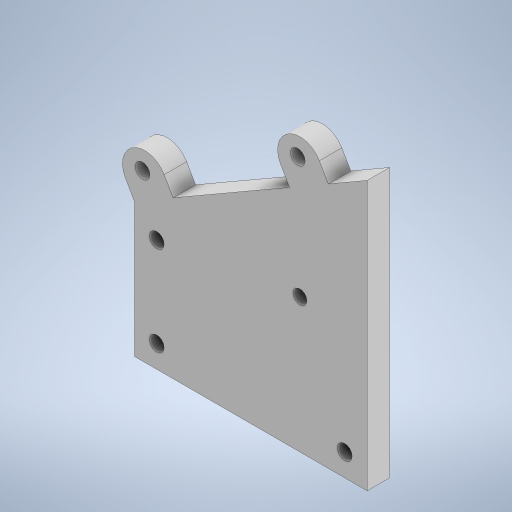
# Autodesk Inventor part: ベースパーツ1
Saved by Autodesk Inventor 2024.3 (Build 283343000, 343)
## iProperties
Created: 2024-10-08
Part Number: ベースパーツ1
Material: 一般
Document SubType Name: Modeling
Designer: hikou
Density: 1 g/cm^3
Appearance: 既定
Author: hikou
Autodesk Inventor part; units mm, degrees
ref_plane "YZ Plane" through (0, 0, 0) normal (1, 0, 0) x (0, 1, 0)
ref_plane "XZ Plane" through (0, 0, 0) normal (0, 1, 0) x (-1, 0, 0)
ref_plane "XY Plane" through (0, 0, 0) normal (0, 0, 1) x (1, 0, 0)
sketch "スケッチ1" plane through (0, 0, 0) normal (0, 0, 1) x (1, 0, 0)
  line L0 (-25.9808, -15) -> (25.9808, -15)
  line L1 (25.9808, -15) -> (25.9808, 15)
  line L2 (25.9808, 15) -> (-25.9808, 15)
  line L3 (-25.9808, 15) -> (-25.9808, -15)
  line L4 (-25.9808, -15) -> (25.9808, 15) construction
  line L5 (25.9808, -15) -> (-25.9808, 15) construction
  line L6 (-25.9808, 15) -> (25.9808, 45)
  line L7 (25.9808, 45) -> (25.9808, 15)
  line L8 (-25.9808, 15) -> (-30.9808, 23.6603)
  line L9 (-30.9808, 23.6603) -> (-22.3205, 28.6603)
  line L10 (-22.3205, 28.6603) -> (-17.3205, 20)
  line L11 (8.6603, 35) -> (3.6603, 43.6603)
  line L12 (3.6603, 43.6603) -> (12.3205, 48.6603)
  line L13 (12.3205, 48.6603) -> (17.3205, 40)
  point P0 (0, 0)
  dimension "d0" = 60
  dimension "d1" = 30
  dimension "d2" = 30
  dimension "d3" = 30
  dimension "d4" = 10
  dimension "d5" = 10
  dimension "d6" = 10
  dimension "d7" = 30
  constraints: 28 end point, 7 perpendicular, 4 point on line, 2 midpoint, 2 parallel, 1 horizontal
  measures "d0" distance of L2.end L6.end
  measures "d1" distance of L6.end L1.end
  measures "d2" angle of L2 L6
  measures "d3" distance of L0.end L1.end
  measures "d4" distance of L2.end L8.end
  measures "d5" distance of L8.end L9.end
  measures "d6" distance of L11.end L12.end
  measures "d7" distance between parallel lines of L10 L11
extrude "押し出し1" add sketch "スケッチ1" along normal mid plane 5
sketch "スケッチ2" plane through (0, 0, 2.5) normal (0, 0, 1) x (1, 0, 0)
  line L0 (-30.9808, 23.6603) -> (-25.9808, 15) projected
  line L1 (-25.9808, 15) -> (-25.9808, -15) projected
  line L2 (-25.9808, -15) -> (25.9808, -15) projected
  line L3 (25.9808, -15) -> (25.9808, 45) projected
  line L4 (25.9808, 45) -> (17.3205, 40) projected
  line L5 (17.3205, 40) -> (12.3205, 48.6603) projected
  line L6 (12.3205, 48.6603) -> (3.6603, 43.6603) projected
  line L7 (3.6603, 43.6603) -> (8.6603, 35) projected
  line L8 (8.6603, 35) -> (-17.3205, 20) projected
  line L9 (-17.3205, 20) -> (-22.3205, 28.6603) projected
  line L10 (-22.3205, 28.6603) -> (-30.9808, 23.6603) projected
  point P0 (0, 0)
  point P1 (-24.1506, 21.8301)
  point P2 (10.4904, 41.8301)
  dimension "d10" = 5
  dimension "d11" = 5
  dimension "d12" = 5
  dimension "d13" = 5
  measures "d10" distance from line of L8 point (-24.151, 21.83)
  measures "d11" distance from line of L8 point (10.49, 41.83)
  measures "d12" distance from line of L9 point (-24.151, 21.83)
  measures "d13" distance from line of point (10.49, 41.83) L7
hole "穴1" at (-24.1506, 21.8301, 2.5) at (10.4904, 41.8301, 2.5) direction (0, 0, -1) diameter 3.3 end through all
sketch "スケッチ3" plane through (0, 0, 2.5) normal (0, 0, 1) x (1, 0, 0)
  circle A0 centre (10.4904, 41.8301) radius 1.65 projected
  circle A1 centre (-24.1506, 21.8301) radius 1.65 projected
  line L0 (-30.9808, 23.6603) -> (-25.9808, 15) projected
  line L1 (-25.9808, 15) -> (-25.9808, -15) projected
  line L2 (-25.9808, -15) -> (25.9808, -15) projected
  line L3 (25.9808, -15) -> (25.9808, 45) projected
  line L4 (25.9808, 45) -> (17.3205, 40) projected
  line L5 (17.3205, 40) -> (12.3205, 48.6603) projected
  line L6 (12.3205, 48.6603) -> (3.6603, 43.6603) projected
  line L7 (3.6603, 43.6603) -> (8.6603, 35) projected
  line L8 (8.6603, 35) -> (-17.3205, 20) projected
  line L9 (-17.3205, 20) -> (-22.3205, 28.6603) projected
  line L10 (-22.3205, 28.6603) -> (-30.9808, 23.6603) projected
  circle A2 centre (-23.6506, 20.9641) radius 5
  circle A3 centre (10.9904, 40.9641) radius 5
  point P0 (0, 0)
  point P1 (6.6603, 38.4641)
  point P2 (15.3205, 43.4641)
  point P3 (-27.9808, 18.4641)
  point P4 (-19.3205, 23.4641)
  dimension "d21" = 10
  dimension "d22" = 1
  dimension "d24" = 4
  dimension "d25" = 10
  dimension "d26" = 1
  dimension "d27" = 4
  constraints: 2 centre point
  measures "d21" diameter of A2
  measures "d22" distance of A1.centre A2.centre
  measures "d24" distance from line of L8 A2.centre
  measures "d25" diameter of A3
  measures "d26" distance of A0.centre A3.centre
  measures "d27" distance from line of L8 A3.centre
extrude "押し出し2" cut sketch "スケッチ3" against normal blind 5 contours L10 L9 A2 L0 | L7 L6 L5 A3
sketch "スケッチ4" plane through (0, 0, 2.5) normal (0, 0, 1) x (1, 0, 0)
  line L0 (-25.9808, -15) -> (25.9808, -15) projected
  line L1 (25.9808, -15) -> (25.9808, 45) projected
  point P0 (0, 0)
  point P1 (10.9808, 15)
  dimension "d30" = 30
  dimension "d31" = 15
  measures "d30" distance from line of L0 point (10.981, 15)
  measures "d31" distance from line of L1 point (10.981, 15)
hole "穴2" at (10.9808, 15, 2.5) direction (0, 0, -1) diameter 3.1 end through all
sketch "スケッチ5" plane through (0, 0, 2.5) normal (0, 0, 1) x (1, 0, 0)
  line L0 (-25.9808, 15) -> (-25.9808, -15) projected
  line L1 (-25.9808, -15) -> (25.9808, -15) projected
  line L2 (25.9808, -15) -> (25.9808, 45) projected
  point P0 (0, 0)
  point P1 (-20.9808, 10)
  point P2 (-20.9808, -10)
  point P3 (20.9808, -10)
  dimension "d39" = 5
  dimension "d40" = 5
  dimension "d41" = 5
  dimension "d42" = 20
  dimension "d43" = 5
  dimension "d44" = 5
  measures "d39" distance from line of L0 point (-20.981, -10)
  measures "d40" distance from line of L1 point (-20.981, -10)
  measures "d41" distance from line of L0 point (-20.981, 10)
  measures "d42" distance of point (-20.981, -10) point (-20.981, 10)
  measures "d43" distance from line of L1 point (20.981, -10)
  measures "d44" distance from line of L2 point (20.981, -10)
hole "穴3" at (-20.9808, 10, 2.5) at (-20.9808, -10, 2.5) at (20.9808, -10, 2.5) direction (0, 0, -1) diameter 3.3 end through all
equation "\"d5\" = d4"
equation "\"d6\" = d4"
equation "\"d11\" = d10"
equation "\"d12\" = d10"
equation "\"d13\" = d10"
equation "\"d27\" = d24"
equation "\"d40\" = d39"
equation "\"d41\" = d39"
equation "\"d43\" = d39"
equation "\"d44\" = d39"
